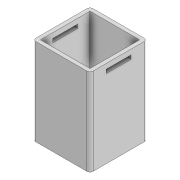
# Autodesk Inventor part: vertical batter holder 4 holes in bottom
Saved by Autodesk Inventor 2020 (Build 240168000, 168)
## iProperties
Created: 2020-01-30
Part Number: vertical batter holder 4 holes in bottom
Material: Generic
Document SubType Name: Modeling
Designer: ball
Density: 1 g/cm^3
Appearance: Default
Author: ball
Autodesk Inventor part; units mm, degrees
ref_plane "YZ Plane" through (0, 0, 0) normal (1, 0, 0) x (0, 1, 0)
ref_plane "XZ Plane" through (0, 0, 0) normal (0, 1, 0) x (-1, 0, 0)
ref_plane "XY Plane" through (0, 0, 0) normal (0, 0, 1) x (1, 0, 0)
sketch "Sketch1" plane through (0, 0, 0) normal (0, 1, 0) x (-1, 0, 0)
  line L0 (25.4, 25.4) -> (-25.4, 25.4)
  line L1 (-25.4, 25.4) -> (-25.4, -25.4)
  line L2 (-25.4, -25.4) -> (25.4, -25.4)
  line L3 (25.4, -25.4) -> (25.4, 25.4)
  line L4 (25.4, 25.4) -> (-25.4, -25.4) construction
  line L5 (-25.4, 25.4) -> (25.4, -25.4) construction
  point P0 (0, 0)
  dimension "d0" = 50.8
  dimension "d1" = 50.8
  constraints: 12 end point, 2 midpoint, 2 parallel, 1 horizontal, 1 perpendicular
  measures "d0" distance of L2.end L1.end
  measures "d1" distance of L1.end L0.end
extrude "Extrusion1" add sketch "Sketch1" along normal blind 5.08
sketch "Sketch2" plane through (0, 5.08, 0) normal (0, 1, 0) x (1, 0, 0)
  line L0 (-25.4, -25.4) -> (25.4, -25.4) projected
  line L1 (-25.4, 25.4) -> (-25.4, -25.4) projected
  line L2 (25.4, -25.4) -> (25.4, 25.4) projected
  line L3 (25.4, 25.4) -> (-25.4, 25.4) projected
  point P0 (0, 0)
  point P1 (-19.05, -19.05)
  point P2 (-19.05, 19.05)
  point P3 (19.05, 19.05)
  point P4 (19.05, -19.05)
  dimension "d4" = 6.35
  dimension "d5" = 6.35
  dimension "d6" = 6.35
  dimension "d7" = 6.35
  dimension "d8" = 6.35
  dimension "d9" = 6.35
  dimension "d10" = 6.35
  dimension "d11" = 6.35
  measures "d4" distance from line of L0 point (-19.05, -19.05)
  measures "d5" distance from line of L1 point (-19.05, -19.05)
  measures "d6" distance from line of L2 point (19.05, -19.05)
  measures "d7" distance from line of L0 point (19.05, -19.05)
  measures "d8" distance from line of L2 point (19.05, 19.05)
  measures "d9" distance from line of L3 point (19.05, 19.05)
  measures "d10" distance from line of L3 point (-19.05, 19.05)
  measures "d11" distance from line of L1 point (-19.05, 19.05)
hole "Hole1" at (-19.05, 5.08, 19.05) at (19.05, 5.08, 19.05) at (19.05, 5.08, -19.05) at (-19.05, 5.08, -19.05) direction (0, -1, 0) diameter 3.937 end through all counterbore diameter 9.525 counterbore depth 2.54
sketch "Sketch3" plane through (0, 0, 0) normal (0, -1, 0) x (1, 0, 0)
  line L0 (-29.21, -25.4) -> (-29.21, 25.4)
  line L1 (-25.4, 25.4) -> (-25.4, -25.4)
  line L2 (-25.4, -25.4) -> (25.4, -25.4)
  line L3 (29.21, -25.4) -> (29.21, -29.21)
  line L4 (29.21, -29.21) -> (-29.21, -29.21)
  line L5 (-29.21, -29.21) -> (-29.21, -25.4)
  line L6 (25.4, -25.4) -> (-25.4, -25.4) projected
  line L7 (29.21, -25.4) -> (29.21, 25.4)
  line L8 (25.4, 25.4) -> (25.4, -25.4)
  line L9 (-25.4, 25.4) -> (25.4, 25.4)
  line L10 (29.21, 25.4) -> (29.21, 29.21)
  line L11 (29.21, 29.21) -> (-29.21, 29.21)
  line L12 (-29.21, 29.21) -> (-29.21, 25.4)
  point P0 (0, 0)
  dimension "d20" = 58.42
  dimension "d21" = 3.81
  dimension "d23" = 58.42
  dimension "d24" = 3.81
  constraints: 24 end point, 6 parallel, 2 horizontal, 2 perpendicular, 2 point on line
  measures "d20" distance of L3.end L4.end
  measures "d21" distance of L3.start L3.end
  measures "d23" distance of L11.end L10.end
  measures "d24" distance of L10.end L10.start
extrude "Extrusion2" add sketch "Sketch3" against normal blind 88.9
fillet "Fillet1" radius 3.175 4 edges at (-29.21, 44.45, 29.21) (-29.21, 44.45, -29.21) (29.21, 44.45, 29.21) (29.21, 44.45, -29.21)
sketch "Sketch4" plane through (-29.21, 0, -26.035) normal (-1, 0, 0) x (0, 0, 1)
  line L0 (13.335, 83.82) -> (38.735, 83.82)
  line L1 (38.735, 83.82) -> (38.735, 80.01)
  line L2 (38.735, 80.01) -> (13.335, 80.01)
  line L3 (13.335, 80.01) -> (13.335, 83.82)
  line L4 (0, 88.9) -> (52.07, 88.9) projected
  line L5 (55.245, 0) -> (55.245, 88.9) projected
  line L6 (-3.175, 88.9) -> (-3.175, 0) projected
  point P0 (26.035, 0)
  dimension "d28" = 25.4
  dimension "d29" = 5.08
  dimension "d30" = 3.81
  dimension "d31" = 16.51
  dimension "d32" = 16.51
  constraints: 8 end point, 2 parallel, 1 horizontal, 1 perpendicular
  measures "d28" distance between parallel lines of L1 L3
  measures "d29" distance between parallel lines of L4 L0
  measures "d30" distance between parallel lines of L2 L0
  measures "d31" distance between parallel lines of L5 L1
  measures "d32" distance between parallel lines of L6 L3
extrude "Extrusion3" cut sketch "Sketch4" against normal through all
equation "\"d6\" = d5"
equation "\"d7\" = d4"
equation "\"d8\" = d6"
equation "\"d9\" = d4"
equation "\"d10\" = d4"
equation "\"d11\" = d5"
body "Solid1"
